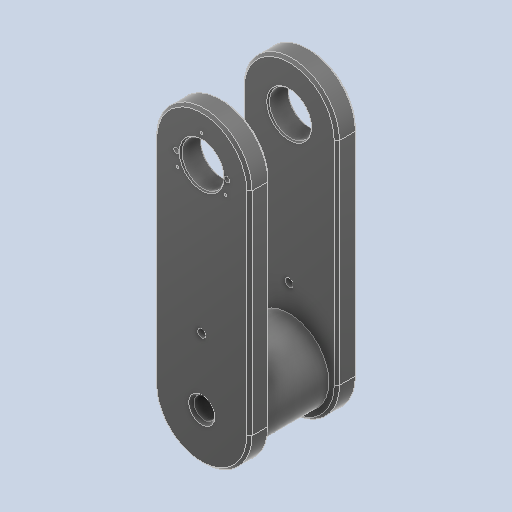
# Autodesk Inventor part: lever_V1
Saved by Autodesk Inventor 2023 (Build 270158000, 158)
## iProperties
Created: 2023-02-13
Part Number: lever_V1
Material: ABS-Kunststoff
Document SubType Name: Modeling
Designer: Mathi
Density: 1.06 g/cm^3
Appearance: Glatt - Weiß
Author: Mathi
Autodesk Inventor part; units mm, degrees
ref_plane "YZ Plane" through (0, 0, 0) normal (1, 0, 0) x (0, 1, 0)
sketch "Skizze1" plane through (0, 0, 0) normal (0, 0, 1) x (1, 0, 0)
  circle A0 centre (0, 0) radius 7.95
  circle A1 centre (0, -80) radius 3.9
  line L0 (0, 0) -> (0, -80) construction
  arc A2 (18, 0) -> (-18, 0) centre (0, 0) ccw
  arc A3 (-18, -80) -> (18, -80) centre (0, -80) ccw
  line L1 (-18, 0) -> (-18, -80)
  line L2 (18, -80) -> (18, 0)
  circle A4 centre (0, -80) radius 15
  circle A5 centre (0, -55) radius 1.5
  circle A6 centre (0, 0) radius 10.45 construction
  line L3 (0, 0) -> (0, 10.45)
  line L4 (-9.05, -5.225) -> (0, 10.45) construction
  line L5 (9.05, -5.225) -> (0, 10.45) construction
  line L6 (-9.05, -5.225) -> (9.05, -5.225) construction
  circle A7 centre (0, 10.45) radius 0.5
  circle A8 centre (-9.05, -5.225) radius 0.5
  circle A9 centre (9.05, -5.225) radius 0.5
  circle A10 centre (0, 0) radius 9.525 construction
  circle A11 centre (-9.525, 0) radius 1
  circle A12 centre (9.525, 0) radius 1
  line L7 (-9.525, 0) -> (0, 0) construction
  line L8 (0, 0) -> (9.525, 0) construction
  circle A13 centre (0, 0) radius 4.1
  circle A14 centre (0, -80) radius 7
  dimension "d0" = 15.9
  dimension "d2" = 36
  dimension "d4" = 80
  dimension "d5" = 30
  dimension "d14" = 7.8
  dimension "d15" = 3
  dimension "d16" = 25
  dimension "d17" = 20.9
  dimension "d18" = 1
  dimension "d19" = 19.05
  dimension "d20" = 2
  dimension "d30" = 8.2
  dimension "d43" = 14
  constraints: 18 end point, 15 centre point, 10 coincident, 9 point on circle, 4 tangent, 3 equal radius, 3 vertical, 2 equal length, 2 horizontal, 1 point on line
  measures "d0" diameter of A0
  measures "d2" diameter of A2
  measures "d4" distance of L0.end L0.start
  measures "d5" diameter of A4
  measures "d14" diameter of A1
  measures "d15" diameter of A5
  measures "d16" distance of A5.centre L0.end
  measures "d17" diameter of A6
  measures "d18" diameter of A7
  measures "d19" diameter of A10
  measures "d20" diameter of A11
  measures "d30" diameter of A13
  measures "d43" diameter of A14
sketch "Skizze2" plane through (0, 0, 0) normal (1, 0, 0) x (0, 1, 0)
  line L0 (18, -20.5) -> (-98, -20.5)
  line L1 (-98, -20.5) -> (-98, -12.5)
  line L2 (-98, -12.5) -> (18, -12.5)
  line L3 (18, -12.5) -> (18, -20.5)
  line L4 (18, 12.5) -> (-98, 12.5)
  line L5 (-98, 12.5) -> (-98, 20.5)
  line L6 (-98, 20.5) -> (18, 20.5)
  line L7 (18, 20.5) -> (18, 12.5)
  line L8 (18, 0) -> (0, 0) projected
  line L9 (-80, 0) -> (-98, 0) projected
  line L10 (-65, 0) -> (-95, 0) projected
  line L11 (18, 12.5) -> (18, 0) construction
  line L12 (18, -12.5) -> (18, 0) construction
  line L13 (-98, 12.5) -> (-98, 0) construction
  line L14 (-65, 12.5) -> (-95, 12.5)
  line L15 (-95, 12.5) -> (-95, -12.5)
  line L16 (-95, -12.5) -> (-65, -12.5)
  line L17 (-65, -12.5) -> (-65, 12.5)
  point P0 (0, 0)
  point P1 (0, 0)
  point P2 (-80, 12.5)
  point P3 (-80, -12.5)
  dimension "d6" = 8
  dimension "d7" = 25
  constraints: 30 end point, 6 parallel, 4 collinear, 4 midpoint, 4 point on line, 3 horizontal, 3 perpendicular
  measures "d6" distance of L6.end L4.start
  measures "d7" distance between parallel lines of L2 L4
ref_plane "Arbeitsebene1" through (0, -80, 12.5) normal (0, 0, 1) x (1, 0, 0)
ref_plane "Arbeitsebene2" through (0, -80, -12.5) normal (0, 0, 1) x (1, 0, 0)
sketch "Skizze3" plane through (0, -80, 12.5) normal (0, 0, 1) x (1, 0, 0)
  arc A0 (-18, 0) -> (18, 0) centre (0, 0) ccw projected
  circle A1 centre (0, 0) radius 3.9 projected
  line L0 (-18, 80) -> (-18, 0) projected
  line L1 (18, 0) -> (18, 80) projected
  circle A2 centre (0, 80) radius 7.95 projected
  arc A3 (18, 80) -> (-18, 80) centre (0, 80) ccw projected
sketch "Skizze4" plane through (0, -80, -12.5) normal (0, 0, 1) x (1, 0, 0)
  point P0 (0, 80)
sketch "Skizze5" plane through (0, -80, -12.5) normal (0, 0, 1) x (1, 0, 0)
  arc A0 (18, 80) -> (-18, 80) centre (0, 80) ccw projected
  line L0 (-18, 80) -> (-18, 0) projected
  line L1 (18, 0) -> (18, 80) projected
  arc A1 (-18, 0) -> (18, 0) centre (0, 0) ccw projected
  circle A2 centre (0, 0) radius 3.9 projected
  circle A3 centre (0, 80) radius 7.95 projected
extrude "Extrusion1" add sketch "Skizze1" along normal blind 8 from surface at 12.5 contours L2 A3 L1 A2 | A4 | A14
extrude "Extrusion2" add sketch "Skizze1" against normal blind 8 from surface at -12.5 contours L2 A3 L1 A2 | A4 | A7 | A8 | A9 | A11 | A12 | A14
extrude "Extrusion3" add sketch "Skizze1" along normal up to surface (25 mm away) from surface at -12.5 contours A4
chamfer "Fase1" distance 1 angle 45 16 edges at (-18, -40, 20.5) (0, 18, 20.5) (18, -40, 20.5) (0, -98, 20.5) (-18, -40, 12.5) (0, 18, 12.5) (18, -40, 12.5) (0, -98, 12.5) (-18, -40, -12.5) (0, 18, -12.5) (18, -40, -12.5) (0, -98, -12.5) (-18, -40, -20.5) (0, 18, -20.5) (18, -40, -20.5) (0, -98, -20.5)
chamfer "Fase2" distance 1 angle 45 2 edges at (-3.9, -80, 20.5) (-3.9, -80, -20.5)
extrude "Extrusion6" add sketch "Skizze1" along normal blind 3 from surface at 12.5 contours A7 | A8 | A9 | A11 | A12
chamfer "Fase5" distance 0.5 angle 45 4 edges at (-7.95, 0, 20.5) (-7.95, 0, 12.5) (-7.95, 0, -12.5) (-7.95, 0, -20.5)
